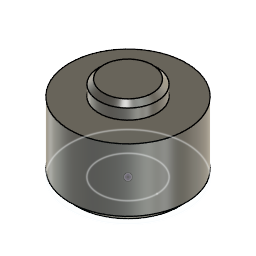
tanto (Autodesk Fusion 360 archive; units mm, degrees)
design "bild nips"
Autodesk Fusion 360 part; units mm, degrees
sketch "Sketch1" plane through (0, 0, 0) normal (0, 0, 1) x (1, 0, 0)
  circle A0 centre (0, 0) radius 2.5
  circle A1 centre (0, 0) radius 1.25
  dimension "d1" = 5
  dimension "d2" = 2.5
  constraint coincident A0.centre A1.centre
  constraint concentric A0 A1
  measures "d1" diameter of A0
  measures "d2" diameter of A1
extrude "Extrude1" add sketch "Sketch1" along normal blind 3
extrude "Extrude2" add sketch "Sketch1" along normal blind 3.65 contours A1
chamfer "Chamfer1" distance 0.3 angle 45 1 edges at (-2.3308, -0.904, 0)
chamfer "Chamfer2" distance 0.2 angle 45 1 edges at (-1.1654, -0.452, 3.65)
equation "d5 = 3 mm + 0.65 mm"
